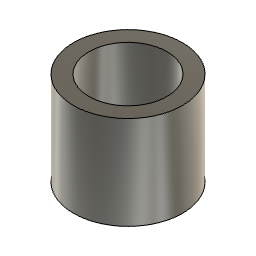
podlozka v1 (Autodesk Fusion 360 design; units mm, degrees)
Autodesk Fusion 360 part; units mm, degrees
sketch "Sketch1" plane through (0, 0, 0) normal (0, 0, 1) x (1, 0, 0)
  circle A0 centre (9.7983, 10.0756) radius 1.25
  circle A1 centre (9.7983, 10.0756) radius 1.75
  dimension "d1" = 2.5
  dimension "d2" = 3.5
  constraint concentric A0 A1
  measures "d1" diameter of A0
  measures "d2" diameter of A1
extrude "Extrude1" add sketch "Sketch1" along normal blind 3
